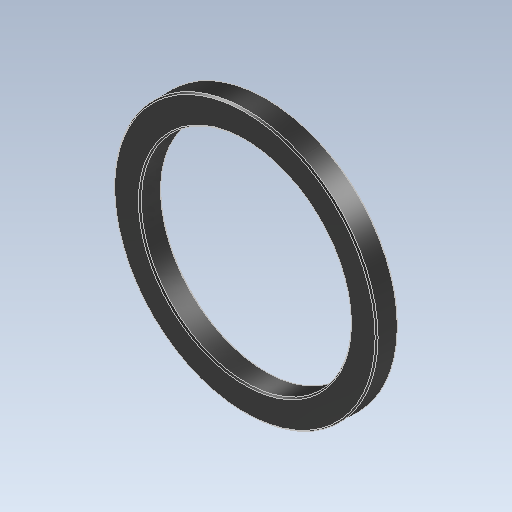
# Autodesk Inventor part: Peça40
Saved by Autodesk Inventor 2021 (Build 250183000, 183)
## iProperties
Created: 2021-07-22
Part Number: Peça40
Material: Genérico
Document SubType Name: Modeling
Designer: Giovanni
Density: 1 g/cm^3
Appearance: Brilhosa - Preta
Mass: 0.13516 g
Surface Area: 3.25175 cm^2
Volume: 0.13516 cm^3
Author: Giovanni
Autodesk Inventor part; units mm, degrees
ref_plane "YZ Plane" through (0, 0, 0) normal (1, 0, 0) x (0, 1, 0)
ref_plane "XZ Plane" through (0, 0, 0) normal (0, 1, 0) x (-1, 0, 0)
ref_plane "XY Plane" through (0, 0, 0) normal (0, 0, 1) x (1, 0, 0)
sketch "Esboço1" plane through (0, 0, 0) normal (0, 0, 1) x (1, 0, 0)
  circle A0 centre (0, 0) radius 7.1
  circle A1 centre (0, 0) radius 8.9
  dimension "d0" = 14.2
  dimension "d1" = 17.8
  constraints: 2 centre point, 2 coincident
  measures "d0" diameter of A0
  measures "d1" diameter of A1
extrude "Extrusão1" add sketch "Esboço1" along normal blind 1.5
chamfer "Chanfro1" distance 0.1 angle 45 4 edges at (-8.9, 0, 1.5) (-8.9, 0, 0) (-7.1, 0, 1.5) (-7.1, 0, 0)
